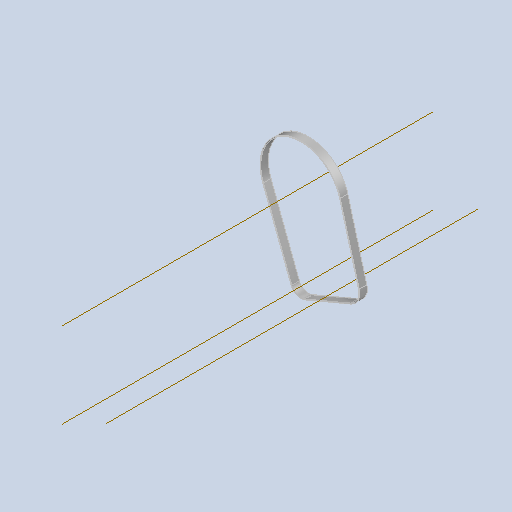
# Autodesk Inventor part: Synchronous Belt
Saved by Autodesk Inventor 2024 (Build 280153000, 153)
## iProperties
CustomPartVersion: 1
Created: 2023-11-23
Part Number: Synchronous Belt
Material: Rubber
Document SubType Name: Modeling
Designer: mb
Density: 1 g/cm^3
Appearance: Rubber - Black - Version 1.1
Author: mb
Autodesk Inventor part; units mm, degrees
sketch "Sketch Path" plane through (0, 0, 0) normal (0, 0, 1) x (1, 0, 0)
  arc A0 (-7.4354, -2.8355) -> (3.0943, -7.3315) centre (0, 0) ccw
  arc A1 (30.7005, 75.4079) -> (-29.7418, 55.6581) centre (0, 67) ccw
  arc A2 (39.275, 7.9388) -> (45.607, 20.9787) centre (34.9977, 18.0732) ccw
  line L0 (39.275, 7.9388) -> (3.0943, -7.3315)
  line L1 (-7.4354, -2.8355) -> (-29.7418, 55.6581)
  line L2 (30.7005, 75.4079) -> (45.607, 20.9787)
  constraints: 6 end point, 6 point on circle, 3 centre point
ref_plane "Cross Section Plane" through (3.0943, -7.3315, 0) normal (0.9213, 0.3888, 0) x (0, 0, 1)
ref_plane "Work Plane2" through (0, 0, 0) normal (-1, 0, 0) x (0, 0, 1)
ref_plane "Work Plane3" through (0, 67, 0) normal (0.3476, -0.9376, 0) x (0, 0, 1)
sketch "Cross Section" plane through (3.0943, -7.3315, 0) normal (0.9213, 0.3888, 0) x (0, 0, 1)
  line L0 (-3, 0.3) -> (3, 0.3)
  line L1 (3, 0.3) -> (3, -0.3)
  line L2 (3, -0.3) -> (-3, -0.3)
  line L3 (-3, -0.3) -> (-3, 0.3)
  line L4 (-3, 0) -> (3, 0) construction
  point P0 (0, 0)
  point P1 (0, 0)
  dimension "d0" = 6
  dimension "d4" = 0.3
  dimension "d5" = 0.3
  constraints: 10 end point, 3 midpoint, 2 parallel, 1 coincident, 1 horizontal, 1 perpendicular, 1 other
  measures "d0" distance between parallel lines of L1 L3
  measures "d4" distance between parallel lines of L2 L4
  measures "d5" distance between parallel lines of L4 L0
sweep "Belt" add profiles "Cross Section" path "Sketch Path"
equation "\"d0\" = da_B"
equation "\"d4\" = da_a"
equation "\"d5\" = da_a2"
equation "\"da_B\" = 6"
equation "\"da_pb\" = 2.5"
equation "\"da_a\" = 0.3"
equation "\"da_S\" = 1.5"
equation "\"da_Beta\" = 20deg"
equation "\"da_Ht\" = 0.7"
equation "\"da_H\" = 1.3"
equation "\"da_a2\" = 0.3"
body "Solid1"
